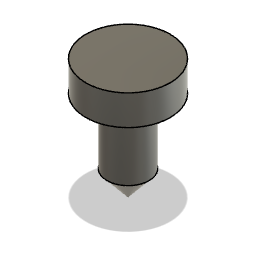
electrode punch tool punch changed v9 (Autodesk Fusion 360 design; units mm, degrees)
Autodesk Fusion 360 part; units mm, degrees
note: some values were not read from the file. Set by a fixed rule: which sketch regions a step uses.
sketch "Sketch1" plane through (0, 0, 0) normal (0, 0, 1) x (1, 0, 0)
  line L0 (0, 0) -> (0, 20)
  line L1 (0, 20) -> (7, 20)
  line L2 (7, 20) -> (7, 15)
  line L3 (7, 15) -> (3.5, 15)
  line L4 (0, 0) -> (0.0013, 0)
  line L5 (0.0013, 0) -> (3.5, 4.1696)
  line L6 (3.5, 4.1696) -> (3.5, 15)
  dimension "d6" = 20
  dimension "d7" = 7
  dimension "d8" = 5
  dimension "d9" = 3.5
  dimension "d13" = 40
  constraint coincident L0.start L4.start
  constraint vertical L0
  constraint perpendicular L0 L1
  constraint perpendicular L1 L2
  constraint perpendicular L2 L3
  constraint perpendicular L0 L4
  constraint perpendicular L3 L6
  measures "d6" distance of L0.start L0.end
  measures "d7" distance of L0.end L1.end
  measures "d8" distance of L1.end L2.end
  measures "d9" distance of L2.end L3.end
  measures "d13" angle of L0 L5
revolve "Revolve2" add sketch "Sketch1" angle 360 about axis through (0, 0, 0) along (0, 1, 0)
